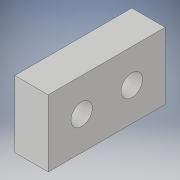
# Autodesk Inventor part: GlyphLiftHolder2
Saved by Autodesk Inventor 2017 (Build 210142000, 142)
## iProperties
Created: 2017-12-29
Part Number: GlyphLiftHolder2
Material: Generic
Document SubType Name: Modeling
Designer: Delta
Density: 1 g/cm^3
Appearance: Default
Author: Delta
Autodesk Inventor part; units mm, degrees
ref_plane "YZ Plane" through (0, 0, 0) normal (1, 0, 0) x (0, 1, 0)
ref_plane "XZ Plane" through (0, 0, 0) normal (0, 1, 0) x (-1, 0, 0)
ref_plane "XY Plane" through (0, 0, 0) normal (0, 0, 1) x (1, 0, 0)
sketch "Sketch1" plane through (0, 0, 0) normal (0, 0, 1) x (1, 0, 0)
  line L0 (0, 0) -> (6.35, 0)
  line L1 (6.35, 0) -> (6.35, 12.7)
  line L2 (6.35, 12.7) -> (0, 12.7)
  line L3 (0, 12.7) -> (0, 0)
  dimension "d0" = 6.35
  dimension "d1" = 12.7
  constraints: 8 end point, 2 parallel, 1 horizontal, 1 perpendicular
  measures "d0" distance of L2.end L1.end
  measures "d1" distance of L1.end L0.end
extrude "Extrusion1" add sketch "Sketch1" along normal blind 22.225
sketch "Sketch2" plane through (0, 0, 0) normal (0, 0, -1) x (-1, 0, 0)
  line L0 (0, 0) -> (-6.35, 0) projected
  line L1 (-3.175, 0) -> (-3.175, 3.175)
  line L2 (-6.35, 12.7) -> (0, 12.7) projected
  line L3 (-3.175, 12.7) -> (-3.175, 9.525)
  dimension "d4" = 3.175
  dimension "d5" = 3.175
  constraints: 4 end point, 2 coincident, 2 midpoint, 2 vertical
  measures "d4" distance of L1.start L1.end
  measures "d5" distance of L3.start L3.end
hole "Hole1" at (3.175, 9.525, 0) at (3.175, 3.175, 0) direction (0, 0, 1) diameter 3.302 depth 4.445 tip angle 118 thread size "8-32 UNC" class "2B" standard "ANSI Unified Screw Threads"
sketch "Sketch3" plane through (0, 0, 0) normal (-1, 0, 0) x (0, 0, 1)
  line L0 (22.225, 0) -> (22.225, 12.7) projected
  line L1 (15.875, 6.35) -> (6.35, 6.35)
  point P0 (0, 0)
  dimension "d14" = 9.525
  constraints: 2 coincident, 2 end point
  measures "d14" distance of L1.start L1.end
hole "Hole2" at (0, 6.35, 15.875) at (0, 6.35, 6.35) direction (1, 0, 0) diameter 4.064 depth 25.4 tip angle 118
body "Solid1"
